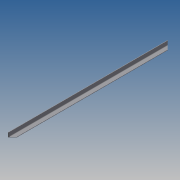
# Autodesk Inventor part: hubRingJigOuter
Saved by Autodesk Inventor 2014 SP1 (Build 180222100, 222)
## iProperties
Created: 2014-12-02
Part Number: hubRingJigOuter
Material: Generic
Document SubType Name: Modeling
Designer: Dave
Density: 1 g/cm^3
Appearance: Default
Author: Dave
Autodesk Inventor part; units mm, degrees
ref_plane "YZ Plane" through (0, 0, 0) normal (1, 0, 0) x (0, 1, 0)
ref_plane "XZ Plane" through (0, 0, 0) normal (0, 1, 0) x (-1, 0, 0)
ref_plane "XY Plane" through (0, 0, 0) normal (0, 0, 1) x (1, 0, 0)
sketch "Sketch1" plane through (0, 0, 0) normal (0, 0, 1) x (1, 0, 0)
  line L0 (0, 0) -> (0, 25.4)
  line L1 (0, 0) -> (25.4, 0)
  line L2 (2.54, 25.4) -> (2.54, 5.715)
  line L3 (5.715, 2.54) -> (25.4, 2.54)
  arc A0 (2.54, 5.715) -> (5.715, 2.54) centre (5.715, 5.715) ccw
  line L4 (0, 25.4) -> (2.54, 25.4)
  line L5 (25.4, 2.54) -> (25.4, 0)
  dimension "d0" = 25.4
  dimension "d1" = 25.4
  dimension "d2" = 2.54
  dimension "d3" = 3.175
  constraints: 12 end point, 3 perpendicular, 2 point on circle, 2 tangent, 1 centre point, 1 parallel, 1 vertical, 1 other
  measures "d0" distance of L0.start L0.end
  measures "d1" distance of L0.start L1.end
  measures "d2" distance between parallel lines of L2 L0
  measures "d3" radius of A0
extrude "Extrusion1" add sketch "Sketch1" along normal blind 914.4
sketch "Sketch2" plane through (0, 0, 0) normal (0, -1, 0) x (1, 0, 0)
  line L0 (25.4, 0) -> (0, 0) projected
  line L1 (25.4, 0) -> (25.4, 914.4) projected
  line L2 (0, 914.4) -> (25.4, 914.4) projected
  line L3 (0, 914.4) -> (25.4, 889)
  line L4 (0, 914.4) -> (60.2005, 914.4) construction
  line L5 (0, 0) -> (25.4, 25.4)
  line L6 (0, 0) -> (85.1364, 0) construction
  dimension "d6" = 45
  dimension "d7" = 45
  constraints: 8 end point, 2 horizontal, 2 point on line
  measures "d6" angle of L3 L4
  measures "d7" angle of L6 L5
extrude "Extrusion2" cut sketch "Sketch2" against normal blind 914.4
sketch "Sketch3" plane through (0, 25.4, 914.4) normal (0, 1, 0) x (1, 0, 0)
  line L0 (2.54, 911.86) -> (0, 914.4) projected
  line L1 (2.54, 911.86) -> (2.54, 2.54) projected
  line L2 (0, 914.4) -> (2.54, 914.4)
  line L3 (2.54, 911.86) -> (2.54, 914.4)
  constraints: 4 end point, 2 perpendicular
extrude "Extrusion3" add sketch "Sketch3" against normal blind 2.54
body "Solid1"
